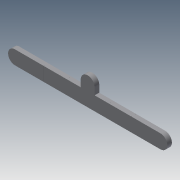
# Autodesk Inventor part: tahlo6_sablona
Saved by Autodesk Inventor 2013 (Build 170138000, 138)
## iProperties
Created: 2013-03-24
Part Number: tahlo6_sablona
Material: Generic
Document SubType Name: Modeling
Designer: idle-rug
Density: 1 g/cm^3
Author: idle-rug
Autodesk Inventor part; units mm, degrees
ref_plane "YZ Plane" through (0, 0, 0) normal (1, 0, 0) x (0, 1, 0)
ref_plane "XZ Plane" through (0, 0, 0) normal (0, 1, 0) x (-1, 0, 0)
ref_plane "XY Plane" through (0, 0, 0) normal (0, 0, 1) x (1, 0, 0)
sketch "Sketch1" plane through (0, 0, 0) normal (0, 1, 0) x (-1, 0, 0)
  line L0 (9, 3) -> (-9, 3)
  line L1 (-9, 3) -> (-9, -3)
  line L2 (-9, -3) -> (9, -3)
  line L3 (9, -3) -> (9, 3)
  line L4 (9, 3) -> (-9, -3) construction
  line L5 (-9, 3) -> (9, -3) construction
  line L6 (-9, -3) -> (-19, -3)
  line L7 (-19, -3) -> (-19, 3)
  line L8 (-19, 3) -> (-9, 3)
  line L9 (-9, 3) -> (-9, -3)
  line L10 (9, -3) -> (19, -3)
  line L11 (19, -3) -> (19, 3)
  line L12 (19, 3) -> (9, 3)
  line L13 (9, 3) -> (9, -3)
  line L14 (-19, -3) -> (-31.5, -3)
  line L15 (-31.5, -3) -> (-31.5, 3)
  line L16 (-31.5, 3) -> (-19, 3)
  line L17 (19, -3) -> (31.5, -3)
  line L18 (31.5, -3) -> (31.5, 3)
  line L19 (31.5, 3) -> (19, 3)
  line L20 (19, 3) -> (19, -3)
  line L21 (-31.5, -3) -> (31.5, -3)
  line L22 (31.5, -3) -> (31.5, 3)
  line L23 (31.5, 3) -> (-31.5, 3)
  line L24 (-31.5, 3) -> (-31.5, -3)
  line L25 (-31.5, -3) -> (31.5, 3) construction
  line L26 (31.5, -3) -> (-31.5, 3) construction
  circle A0 centre (-31.5, 0) radius 3
  circle A1 centre (31.5, 0) radius 3
  line L27 (-9, 3) -> (-9, -3)
  line L28 (-9, -3) -> (-9.01, -3)
  line L29 (-9.01, -3) -> (-9.01, 3)
  line L30 (-9.01, 3) -> (-9, 3)
  line L31 (-19, 3) -> (-19.01, 3)
  line L32 (-19.01, 3) -> (-19.01, -3)
  line L33 (-19.01, -3) -> (-19, -3)
  line L34 (-19, -3) -> (-19, 3)
  line L35 (9, 3) -> (9, -3)
  line L36 (9, -3) -> (9.01, -3)
  line L37 (9.01, -3) -> (9.01, 3)
  line L38 (9.01, 3) -> (9, 3)
  line L39 (19, -3) -> (19, 3)
  line L40 (19, 3) -> (19.01, 3)
  line L41 (19.01, 3) -> (19.01, -3)
  line L42 (19.01, -3) -> (19, -3)
  circle A2 centre (-31.5, 0) radius 0.005
  circle A3 centre (31.5, 0) radius 0.005
  point P0 (0, 0)
  dimension "d0" = 18
  dimension "d1" = 6
  dimension "d2" = 10
  dimension "d3" = 10
  dimension "d4" = 12.5
  dimension "d5" = 12.5
  dimension "d6" = 6
  dimension "d7" = 6
  dimension "d8" = 0.01
  dimension "d9" = 6
  dimension "d10" = 0.01
  dimension "d11" = 6
  dimension "d12" = 0.01
  dimension "d13" = 6
  dimension "d14" = 0.01
  dimension "d15" = 6
  dimension "d16" = 0.01
  dimension "d17" = 0.01
  constraints: 86 end point, 12 parallel, 8 point on line, 7 perpendicular, 6 collinear, 6 horizontal, 6 midpoint, 4 centre point, 2 coincident
  measures "d0" distance of L2.end L1.end
  measures "d1" distance of L1.end L0.end
  measures "d2" distance of L7.end L8.end
  measures "d3" distance of L12.end L11.end
  measures "d4" distance of L15.end L16.end
  measures "d5" distance of L19.end L18.end
  measures "d6" diameter of A0
  measures "d7" diameter of A1
  measures "d8" distance of L1.end L28.end
  measures "d9" distance of L28.end L29.end
  measures "d10" distance of L16.end L31.end
  measures "d11" distance of L31.end L32.end
  measures "d12" distance of L2.end L36.end
  measures "d13" distance of L36.end L37.end
  measures "d14" distance of L19.end L40.end
  measures "d15" distance of L40.end L41.end
  measures "d16" diameter of A2
  measures "d17" diameter of A3
extrude "Extrusion1" add sketch "Sketch1" along normal blind 2 contours L3 L2 L1 L0 | L12 L11 L10 L37 | L29 L6 L7 L8 | L19 A1 L17 L41 | L32 L14 A0 L16 | A1 L18 | L18 A1 | A0 L15 | L15 A0
sketch "Sketch2" plane through (0, 0, 0) normal (0, -1, 0) x (1, 0, 0)
  line L0 (-9, 3) -> (9, 3) projected
  line L1 (-9, -3) -> (-9, 3) projected
  line L2 (9, -3) -> (-9, -3) projected
  line L3 (9, 3) -> (9, -3) projected
  line L4 (0, -3) -> (0, 0)
  circle A0 centre (0, 0) radius 1.5
  line L5 (0, 1.5) -> (0, 4.5)
  line L6 (0, 4.5) -> (0, 6)
  circle A1 centre (0, 6) radius 1.5
  line L7 (0, 6) -> (0, 9)
  circle A2 centre (0, 6) radius 3
  line L8 (-3, 6) -> (-3, 3)
  line L9 (3, 6) -> (3, 3)
  dimension "d21" = 3
  dimension "d20" = 3
  dimension "d22" = 3
  dimension "d23" = 1.5
  dimension "d24" = 3
  dimension "d25" = 3
  constraints: 12 end point, 3 coincident, 3 collinear, 3 point on circle, 2 centre point, 2 perpendicular, 2 point on line, 2 tangent, 1 midpoint, 1 parallel, 1 vertical alignment, 2 other
  measures "d20" distance of L4.start L4.end
  measures "d22" distance of L5.start L5.end
  measures "d23" distance of L5.end L6.end
  measures "d24" diameter of A1
  measures "d25" distance of L7.start L7.end
extrude "Extrusion2" add sketch "Sketch2" against normal blind 2 contours L8 A2 L0 | A2 L9 L0 | A2 L7 A1 L5 | L5 A1 L7 A2 | A0
sketch "Sketch3" plane through (0, 0, 0) normal (0, -1, 0) x (1, 0, 0)
  circle A0 centre (0, 6) radius 1.5 projected
  arc A1 (3, 6) -> (-3, 6) centre (0, 6) ccw projected
  circle A2 centre (0, 0) radius 0.005
  circle A3 centre (0, 6) radius 0.005
  dimension "d28" = 0.01
  dimension "d29" = 0.01
  constraints: 2 centre point, 2 coincident
  measures "d28" diameter of A2
  measures "d29" diameter of A3
extrude "Extrusion3" cut sketch "Sketch3" against normal blind 2
sketch "Sketch4" plane through (0, 0, 0) normal (0, -1, 0) x (1, 0, 0)
  circle A0 centre (0, 6) radius 1.5 projected
  arc A1 (3, 6) -> (-3, 6) centre (0, 6) ccw projected
  circle A2 centre (0, 6) radius 0.005
  dimension "d32" = 0.01
  constraints: 1 centre point, 1 coincident
  measures "d32" diameter of A2
extrude "Extrusion4" add sketch "Sketch4" against normal blind 2
sketch "Sketch5" plane through (0, 0, 0) normal (0, -1, 0) x (1, 0, 0)
  circle A0 centre (0, 0) radius 0.005 projected
  arc A1 (3, 6) -> (-3, 6) centre (0, 6) ccw projected
  circle A2 centre (0, 6) radius 0.05
  circle A3 centre (0, 0) radius 0.05
  dimension "d35" = 0.1
  dimension "d36" = 0.1
  constraints: 2 centre point, 2 coincident
  measures "d35" diameter of A2
  measures "d36" diameter of A3
extrude "Extrusion5" cut sketch "Sketch5" against normal blind 2 contours A0 | A2 | A3
sketch "Sketch6" plane through (0, 0, 0) normal (0, -1, 0) x (1, 0, 0)
  arc A0 (-31.5, 3) -> (-31.5, -3) centre (-31.5, 0) ccw projected
  circle A1 centre (-31.5, 0) radius 0.05
  point P0 (0, 0)
  dimension "d39" = 0.1
  constraints: 1 centre point, 1 coincident
  measures "d39" diameter of A1
extrude "Extrusion6" cut sketch "Sketch6" against normal blind 2
sketch "Sketch7" plane through (0, 0, 0) normal (0, -1, 0) x (1, 0, 0)
  arc A0 (31.5, -3) -> (31.5, 3) centre (31.5, 0) ccw projected
  circle A1 centre (31.5, 0) radius 0.05
  point P0 (0, 0)
  dimension "d42" = 0.1
  constraints: 1 centre point, 1 coincident
  measures "d42" diameter of A1
extrude "Extrusion7" cut sketch "Sketch7" against normal blind 2
body "Solid1"
